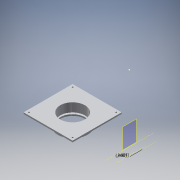
# Autodesk Inventor part: TrapAdapter
Saved by Autodesk Inventor 2019 (Build 230136000, 136)
## iProperties
Created: 2018-12-17
Part Number: TrapAdapter
Material: ABS Plastic
Document SubType Name: Modeling
Designer: assman
Density: 1.06 g/cm^3
Appearance: Smooth - White
Author: assman
Autodesk Inventor part; units mm, degrees
ref_plane "Work Plane1" through (-148.5253, -91.81, -70.5943) normal (0, -1, 0) x (1, 0, 0)
sketch "Sketch6" plane through (-148.5253, -91.81, -70.5943) normal (0, -1, 0) x (1, 0, 0)
  line L0 (182.9917, 36.1279) -> (114.0589, 36.1279) projected
  line L1 (182.9917, 105.0607) -> (182.9917, 36.1279) projected
  line L2 (114.0589, 36.1279) -> (114.0589, 105.0607) projected
  line L3 (114.0589, 105.0607) -> (182.9917, 105.0607) projected
  circle A0 centre (179.1553, 101.2243) radius 1 projected
  circle A1 centre (117.8953, 101.2243) radius 1 projected
  circle A2 centre (117.8953, 39.9643) radius 1 projected
  circle A3 centre (179.1553, 39.9643) radius 1 projected
  point P0 (148.5253, 70.5943)
extrude "Extrusion1" add sketch "Sketch6" along normal blind 2
ref_plane "Work Plane3" through (-148.5253, -93.81, -70.5943) normal (0, -1, 0) x (1, 0, 0)
sketch "Sketch7" plane through (-148.5253, -93.81, -70.5943) normal (0, -1, 0) x (1, 0, 0)
  circle A0 centre (148.5253, 70.5943) radius 17.272
  dimension "d3" = 34.544
  constraints: 1 centre point, 1 coincident
  measures "d3" diameter of A0
extrude "Extrusion2" cut sketch "Sketch7" against normal blind 2
ref_plane "Work Plane2" through (-148.5253, -93.81, -70.5943) normal (0, -1, 0) x (1, 0, 0)
sketch "Sketch8" plane through (-148.5253, -93.81, -70.5943) normal (0, -1, 0) x (1, 0, 0)
  circle A0 centre (148.5253, 70.5943) radius 19.272
  circle A1 centre (148.5253, 70.5943) radius 17.272 projected
  dimension "d6" = 2
  constraints: 1 centre point, 1 coincident
  measures "d6" radial gap between concentric circles of A1 A0
extrude "Extrusion3" add sketch "Sketch8" along normal blind 10.3076
sketch "Sketch9" plane through (-148.5253, -93.81, -70.5943) normal (0, -1, 0) x (1, 0, 0)
  arc A0 (160.2004, 63.2971) -> (137.9644, 32.6515) centre (152.0021, 45.8559) ccw projected
  circle A1 centre (148.5253, 70.5943) radius 19.272 projected
  arc A2 (161.3025, 87.6014) -> (127.2533, 70.5943) centre (148.5253, 70.5943) ccw
  line L0 (129.2533, 70.5943) -> (127.2533, 70.5943)
  line L1 (161.3025, 87.6014) -> (160.1012, 86.0024)
  dimension "d9" = 2
  dimension "d10" = 1.599
  constraints: 4 end point, 2 point on circle, 1 centre point, 1 horizontal, 1 line through centre, 5 other
  measures "d10" vertical distance of L1.start L1.end
ref_plane "Work Plane4" through (79.84, -63.33, -9.91) normal (-1, 0, 0) x (0, 1, 0)
sketch "Sketch10" plane through (79.84, -63.33, -9.91) normal (-1, 0, 0) x (0, 1, 0)
  line L0 (-30.48, -44.3764) -> (-30.48, 24.5564) construction
  line L1 (-40.7876, 9.362) -> (-40.7876, -29.182) construction
  line L2 (-42.7826, 28.0328) -> (-42.7826, -4.4435) construction
  point P0 (63.33, -9.91)
  dimension "d11" = 10.3076
  dimension "d12" = 12.3026
  measures "d11" distance between parallel lines of L0 L1
  measures "d12" distance between parallel lines of L0 L2
extrude "Extrusion4" add sketch "Sketch9" along normal blind 12.4936 contours A1 L0 A2 L1
sketch "Sketch11" plane through (-148.5253, -106.3036, -70.5943) normal (0, -1, 0) x (1, 0, 0)
  arc A0 (236.18, 74.3245) -> (238.4751, 66.3206) centre (237.3276, 70.3226) ccw construction
  line L0 (236.18, 74.3245) -> (189.5181, 60.9444) construction
  arc A1 (160.2004, 63.2971) -> (189.5181, 60.9444) centre (177.9908, 101.1449) ccw construction
  arc A2 (160.2004, 63.2971) -> (137.9644, 32.6515) centre (152.0021, 45.8559) ccw construction
  line L1 (136.5076, 31.2812) -> (137.9644, 32.6515) construction
  arc A3 (136.5076, 31.2812) -> (169.8778, 34.3252) centre (152.0021, 45.8559) ccw construction
  arc A4 (172.0656, 37.3886) -> (169.8778, 34.3252) centre (203.3405, 12.74) ccw construction
  line L2 (170.4948, 38.6266) -> (172.0656, 37.3886) construction
  arc A5 (191.8132, 52.9405) -> (170.4948, 38.6266) centre (203.3405, 12.74) ccw construction
  line L3 (191.8132, 52.9405) -> (238.4751, 66.3206) construction
  line L4 (129.2533, 70.5943) -> (127.2533, 70.5943) construction
  line L5 (129.2533, 70.5943) -> (165.4777, 70.5943) construction
  circle A6 centre (148.5253, 70.5943) radius 17.272 construction
  line L6 (148.5253, 87.8663) -> (148.5253, 53.3223) construction
  circle A7 centre (148.5253, 70.5943) radius 17.272 construction
  circle A8 centre (148.5253, 70.5943) radius 19.272 construction
  circle A9 centre (148.5253, 70.5943) radius 21.272
  dimension "d15" = 42.544
  constraints: 4 end point, 2 centre point, 2 coincident, 2 point on circle, 1 horizontal, 1 vertical, 2 other
  measures "d15" diameter of A9
extrude "Extrusion5" add sketch "Sketch11" along normal blind 2
sketch "Sketch12" plane through (0, -108.3036, 0) normal (0, -1, 0) x (1, 0, 0)
  circle A0 centre (0, 0) radius 17.2734 projected
extrude "Extrusion6" cut sketch "Sketch12" against normal blind 2
body "Solid1"
